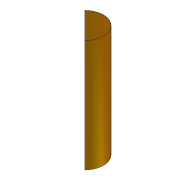
# Autodesk Inventor part: kaptonheater_OmegaKHLV102
Saved by Autodesk Inventor 2014 SP1 (Build 180222100, 222)
## iProperties
Created: 2013-03-29
Part Number: kaptonheater_OmegaKHLV102
Material: Acetal Resin, Black
Document SubType Name: Modeling
Designer: Robert Davis
Density: 1.425 g/cm^3
Mass: 0.185786 g
Surface Area: 26.2274 cm^2
Volume: 0.130376 cm^3
Appearance: Orange (Dark)
Author: Robert Davis
Autodesk Inventor part; units mm, degrees
ref_plane "YZ Plane" through (0, 0, 0) normal (1, 0, 0) x (0, 1, 0)
ref_plane "XZ Plane" through (0, 0, 0) normal (0, 1, 0) x (-1, 0, 0)
ref_plane "XY Plane" through (0, 0, 0) normal (0, 0, 1) x (1, 0, 0)
sketch "Sketch1" plane through (0, 0, 0) normal (0, 0, 1) x (1, 0, 0)
  arc A0 (5.8336, -5.8336) -> (-5.8336, 5.8336) centre (0, 0) ccw
  line L0 (-5.8336, 5.8336) -> (0, 0) construction
  line L1 (0, 0) -> (5.8336, -5.8336) construction
  line L2 (0, 0) -> (0, -21.6093) construction
  arc A1 (5.9043, -5.9043) -> (-5.9043, 5.9043) centre (0, 0) ccw
  line L3 (-5.9043, 5.9043) -> (-5.8336, 5.8336)
  line L4 (5.9043, -5.9043) -> (5.8336, -5.8336)
  dimension "d0" = 8.25
  dimension "d1" = 180
  dimension "d2" = 45
  dimension "d3" = 0.1
  constraints: 10 end point, 4 point on circle, 2 centre point, 2 coincident, 2 collinear, 1 vertical
  measures "d0" radius of A0
  measures "d1" angle of L1 L0
  measures "d2" angle of L1 L2
  measures "d3" distance of L3.start L0.start
extrude "Extrusion1" add sketch "Sketch1" along normal mid plane 50
body "Solid1"
